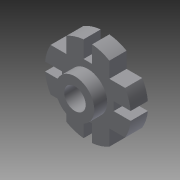
# Autodesk Inventor part: HW 2 Part 5
Saved by Autodesk Inventor 2015 (Build 190159000, 159)
## iProperties
Created: 2016-01-24
Part Number: HW 2 Part 5
Material: Generic
Document SubType Name: Modeling
Designer: Melissa
Density: 1 g/cm^3
Appearance: Default
Author: Melissa
Autodesk Inventor part; units mm, degrees
ref_plane "YZ Plane" through (0, 0, 0) normal (1, 0, 0) x (0, 1, 0)
ref_plane "XZ Plane" through (0, 0, 0) normal (0, 1, 0) x (-1, 0, 0)
ref_plane "XY Plane" through (0, 0, 0) normal (0, 0, 1) x (1, 0, 0)
sketch "Sketch1" plane through (0, 0, 0) normal (0, 0, 1) x (1, 0, 0)
  circle A0 centre (0, 0) radius 63.5
  circle A1 centre (0, 0) radius 15.875
  dimension "d0" = 127
  dimension "d1" = 31.75
  constraints: 2 centre point, 2 coincident
  measures "d0" diameter of A0
  measures "d1" diameter of A1
extrude "Extrusion1" add sketch "Sketch1" along normal blind 25.4
sketch "Sketch2" plane through (0, 0, 25.4) normal (0, 0, 1) x (1, 0, 0)
  circle A0 centre (0, 0) radius 28.575
  circle A1 centre (0, 0) radius 15.875
  dimension "d4" = 57.15
  dimension "d5" = 31.75
  constraints: 2 centre point, 2 coincident
  measures "d4" diameter of A0
  measures "d5" diameter of A1
extrude "Extrusion2" add sketch "Sketch2" along normal blind 19.05
sketch "Sketch3" plane through (0, 0, 25.4) normal (0, 0, 1) x (1, 0, 0)
  line L0 (-38.1, -38.1) -> (38.1, -38.1)
  line L1 (38.1, -38.1) -> (38.1, 38.1)
  line L2 (38.1, 38.1) -> (-38.1, 38.1)
  line L3 (-38.1, 38.1) -> (-38.1, -38.1)
  line L4 (-6.35, 38.1) -> (-6.35, 66.3374)
  line L5 (-6.35, 38.1) -> (6.35, 38.1)
  line L6 (6.35, 38.1) -> (6.35, 66.3374)
  line L7 (6.35, 66.3374) -> (-6.35, 66.3374)
  line L8 (-38.1, -6.35) -> (-66.3374, -6.35)
  line L9 (-38.1, 6.35) -> (-66.3374, 6.35)
  line L10 (-66.3374, 6.35) -> (-66.3374, -6.35)
  line L11 (-6.35, -38.1) -> (-6.35, -66.3374)
  line L12 (6.35, -38.1) -> (6.35, -66.3374)
  line L13 (6.35, -66.3374) -> (-6.35, -66.3374)
  line L14 (38.1, 6.35) -> (66.3374, 6.35)
  line L15 (38.1, -6.35) -> (66.3374, -6.35)
  line L16 (66.3374, 6.35) -> (66.3374, -6.35)
  line L17 (-38.1, -6.35) -> (-38.1, 6.35)
  line L18 (-6.35, -38.1) -> (6.35, -38.1)
  line L19 (38.1, -6.35) -> (38.1, 6.35)
  point P0 (0, 0)
  dimension "d8" = 76.2
  constraints: 40 end point, 4 perpendicular, 3 vertical, 2 collinear, 2 parallel, 2 point on line, 1 horizontal
  measures "d8" distance of L2.end L1.end
extrude "Extrusion3" cut sketch "Sketch3" against normal through all contours L0 L12 L13 L11 | L8 L10 L9 L3 | L1 L14 L16 L15 | L4 L7 L6 L2
sketch "Sketch4" plane through (0, 0, 25.4) normal (0, 0, 1) x (1, 0, 0)
  line L0 (31.75, 31.75) -> (130.2144, 31.75)
  line L1 (63.1817, -6.35) -> (38.1, -6.35) projected
  line L2 (0, 0) -> (95.3725, 0)
  line L3 (0, 0) -> (0, 66.6)
  line L4 (31.75, 31.75) -> (31.75, 99.3108)
  line L5 (31.75, -31.75) -> (130.2144, -31.75)
  line L6 (31.75, -31.75) -> (31.75, -99.3108)
  line L7 (31.75, 99.3108) -> (130.2144, 31.75)
  line L8 (31.75, -99.3108) -> (130.2144, -31.75)
  line L9 (-31.75, 31.75) -> (-130.2144, 31.75)
  line L10 (-31.75, 31.75) -> (-31.75, 99.3108)
  line L11 (-31.75, -31.75) -> (-31.75, -99.3108)
  line L12 (-31.75, -31.75) -> (-130.2144, -31.75)
  line L13 (-31.75, 99.3108) -> (-130.2144, 31.75)
  line L14 (-31.75, -99.3108) -> (-130.2144, -31.75)
  dimension "d18" = 31.75
  dimension "d19" = 31.75
  constraints: 28 end point, 9 symmetric about line, 2 horizontal, 2 vertical
  measures "d18" distance between parallel lines of L2 L0
  measures "d19" distance between parallel lines of L4 L3
extrude "Extrusion4" cut sketch "Sketch4" against normal through all
body "Solid1"
